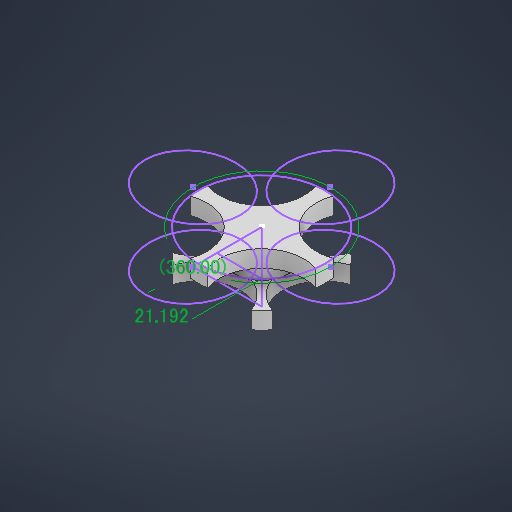
# Autodesk Inventor part: Part1
Saved by Autodesk Inventor 2026 (Build 300175000, 175)
## iProperties
Created: 2025-10-14
Part Number: Part1
Material: 一般
Document SubType Name: Modeling
Designer: masak
Density: 1 g/cm^3
Appearance: 既定
Author: masak
Autodesk Inventor part; units mm, degrees
ref_plane "YZ Plane" through (0, 0, 0) normal (1, 0, 0) x (0, 1, 0)
ref_plane "XZ Plane" through (0, 0, 0) normal (0, 1, 0) x (-1, 0, 0)
ref_plane "XY Plane" through (0, 0, 0) normal (0, 0, 1) x (1, 0, 0)
sketch "スケッチ1" plane through (0, 0, 0) normal (0, 1, 0) x (-1, 0, 0)
  circle A0 centre (0, 0) radius 25
  circle A1 centre (0, 0) radius 30
  dimension "d0" = 50
  dimension "d1" = 60
  constraints: 2 centre point, 2 coincident
  measures "d0" diameter of A0
  measures "d1" diameter of A1
extrude "押し出し1" add sketch "スケッチ1" along normal blind 8 contours A0 | A1
sketch "スケッチ2" plane through (0, 8, 0) normal (0, 1, 0) x (1, 0, 0)
  circle A0 centre (0, 0) radius 30 projected
  line L0 (0, -30) -> (-30, 0)
  line L1 (-30, 0) -> (0, 30)
  line L2 (0, 30) -> (30, 0)
  line L3 (0, -30) -> (30, 0)
  circle A1 centre (0, 0) radius 30
  circle A2 centre (0, 0) radius 25
  circle A3 centre (-23, 23) radius 20
  circle A4 centre (-23, -23) radius 20
  circle A5 centre (23, -23) radius 20
  circle A6 centre (23, 23) radius 20
  point P0 (-4.1593, 29.7103)
  point P1 (-29.7103, 4.1593)
  dimension "d5" = 50
  dimension "d8" = 23
  dimension "d9" = 23
  dimension "d13" = 360
  dimension "d29" = 40
  constraints: 8 end point, 6 centre point, 3 point on circle, 2 coincident, 1 concentric, 9 other
  measures "d5" diameter of A2
  measures "d8" horizontal distance of A3.centre point (0, 0)
  measures "d9" horizontal distance of point (0, 0) A3.centre
  measures "d29" diameter of A3
extrude "押し出し2" cut sketch "スケッチ2" against normal blind 10 contours A6 L2 A2 A0 | A0 A6 | A5 A0 | A0 A5 L3 A2 | A6 A2 L2 | L3 A2 A5 | A2 A6 L2 | L2 A2 | A2 L3 | L3 A2 A5 | L2 A2 A6 | A5 A2 L3 | A3 L1 A2 A0 | A0 A3 | A3 A2 L1 | A4 A0 | A0 A4 L0 A2 | L0 A2 A4 | A3 A2 L1 | A2 L0 A4 | L1 A2 | A2 L0 | L1 A2 A3 | A4 A2 L0
sketch "スケッチ3" plane through (0, 8, 0) normal (0, 1, 0) x (1, 0, 0)
  line L0 (0, -0.0001) -> (0, -29.9755)
  circle A0 centre (-0.0169, 0.0244) radius 30
  line L1 (0, -0.0001) -> (32.5269, -32.527)
  line L2 (32.5269, -32.527) -> (0, -32.527)
  line L3 (21.1924, -21.1926) -> (0, -21.1926)
  ellipse E0 centre (0, -32.527) end of major axis (20.2314, -32.527) minor radius 22.6164
  ellipse E1 centre (32.5345, 0.0414) end of major axis (32.5345, 20.2728) minor radius 22.6164
  ellipse E2 centre (-0.0339, 32.5759) end of major axis (-20.2653, 32.5759) minor radius 22.6164
  ellipse E3 centre (-32.5684, 0.0075) end of major axis (-32.5684, -20.2239) minor radius 22.6164
  point P0 (0, 0)
  point P1 (-4.1509, 30.0937)
  point P2 (-30.9256, 3.319)
  dimension "d50" = 21.1925
  dimension "d51" = 360
  constraints: 8 end point, 3 point on line, 2 centre point, 2 coincident, 16 other
  measures "d50" distance of L3.start L3.end
sketch "スケッチ4" plane through (0, 0, 0) normal (0, -1, 0) x (1, 0, 0)
  circle A0 centre (0, 0) radius 12.5
  dimension "d15" = 25
  constraints: 1 centre point, 1 coincident
  measures "d15" diameter of A0
extrude "押し出し3" add sketch "スケッチ4" along normal blind 5
sketch "スケッチ5" plane through (0, -5, 0) normal (0, -1, 0) x (1, 0, 0)
  circle A0 centre (0, 0) radius 30
  dimension "d18" = 60
  constraints: 1 centre point, 1 coincident
  measures "d18" diameter of A0
extrude "押し出し4" add sketch "スケッチ5" along normal blind 8
sketch "スケッチ6" plane through (0, -13, 0) normal (0, -1, 0) x (1, 0, 0)
  line L0 (0.0169, -0.0245) -> (0.0169, -30)
  circle A0 centre (0, 0) radius 30 projected
  line L1 (0.0169, -0.0245) -> (32.5438, -32.5514)
  line L2 (32.5438, -32.5514) -> (0.0169, -32.5514)
  line L3 (21.2094, -21.217) -> (0.0169, -21.217)
  ellipse E0 centre (0.0169, -32.5514) end of major axis (20.2483, -32.5514) minor radius 22.6164
  ellipse E1 centre (32.5514, 0.0169) end of major axis (32.5514, 20.2483) minor radius 22.6164
  ellipse E2 centre (-0.0169, 32.5514) end of major axis (-20.2483, 32.5514) minor radius 22.6164
  ellipse E3 centre (-32.5514, -0.0169) end of major axis (-32.5514, -20.2483) minor radius 22.6164
  point P0 (-3.3011, 29.5474)
  point P1 (-30.0758, 2.7727)
  dimension "d43" = 21.1925
  dimension "d46" = 360
  constraints: 8 end point, 3 point on line, 2 centre point, 2 coincident, 2 perpendicular, 2 point on circle, 1 vertical, 13 other
  measures "d43" distance of L3.start L3.end
extrude "押し出し5" cut sketch "スケッチ6" against normal blind 8 contours E0 L3 L0 | L0 A0 E0 | L3 E0 A0 L0 | A0 E0 | E1 A0 | A0 E1 | E3 A0 | A0 E3 | E2 A0 | A0 E2
